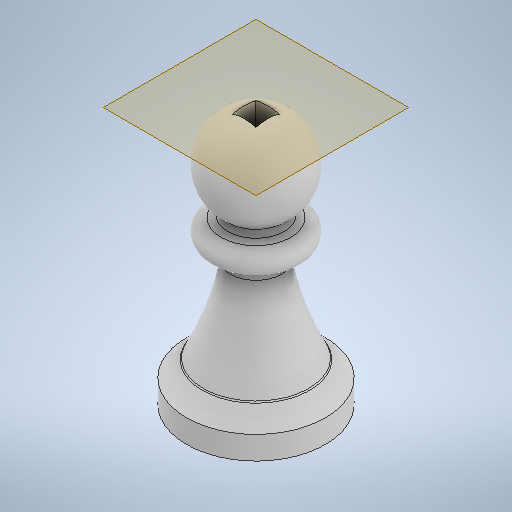
# Autodesk Inventor part: PawnUntagged
Saved by Autodesk Inventor 2025.2 (Build 292293000, 293)
## iProperties
Created: 2025-02-26
Part Number: PawnUntagged
Material: Generic
Document SubType Name: Modeling
Designer: Marcu
Density: 1 g/cm^3
Appearance: Default
Author: Marcu
Autodesk Inventor part; units mm, degrees
ref_plane "YZ Plane" through (0, 0, 0) normal (1, 0, 0) x (0, 1, 0)
ref_plane "XY Plane" through (0, 0, 0) normal (0, 0, 1) x (1, 0, 0)
sketch "Sketch1" plane through (0, 0, 0) normal (1, 0, 0) x (0, 1, 0)
  line L0 (4, 0) -> (4, 2.5)
  line L1 (4, 2.5) -> (0.0049, 2.5)
  line L2 (0.0049, 2.5) -> (0.0049, 15)
  line L3 (0.0049, 15) -> (5.0049, 15)
  line L4 (5.0049, 15) -> (8.4215, 11.5834)
  arc A0 (8.6928, 11.3905) -> (27.0718, 5.4521) centre (39.1985, 74.3936) ccw
  line L5 (30.0049, 7.9143) -> (30.0049, 7.5)
  line L6 (32.5049, 10) -> (32.5049, 10)
  line L7 (35.0049, 7.5) -> (35.0049, 7.5)
  arc A1 (55.0049, 0) -> (37.0518, 6.0621) centre (45.0049, 0) ccw
  line L8 (4, 0) -> (55.0049, 0)
  arc A2 (35.0049, 7.5) -> (35.4243, 6.1139) centre (37.5049, 7.5) ccw
  arc A3 (35.0049, 7.5) -> (32.5049, 10) centre (32.5049, 7.5) ccw
  arc A4 (32.5049, 10) -> (30.0049, 7.5) centre (32.5049, 7.5) ccw
  arc A5 (27.0718, 5.4521) -> (30.0049, 7.9143) centre (27.5049, 7.9143) ccw
  arc A6 (35.4243, 6.1139) -> (37.0518, 6.0621) centre (36.2565, 6.6683) ccw
  arc A7 (8.4215, 11.5834) -> (8.6928, 11.3905) centre (9.1286, 12.2905) ccw
  point P0 (0, 0)
  point P1 (0, 0)
  point P2 (8.5404, 11.4645)
  point P3 (30.0049, 5)
  point P4 (30.0049, 10)
  point P5 (35.0049, 10)
  point P6 (35.0049, 5)
  dimension "d0" = 4
  dimension "d1" = 2.5
  dimension "d2" = 15
  dimension "d3" = 5
  dimension "d4" = 5
  dimension "d5" = 135
  dimension "d6" = 70
  dimension "d7" = 5
  dimension "d8" = 5
  dimension "d9" = 5
  dimension "d10" = 2.5
  dimension "d11" = 1
  dimension "d12" = 1
  constraints: 18 end point, 18 point on circle, 11 tangent, 8 centre point, 7 point on line, 3 equal radius, 3 perpendicular, 2 horizontal, 2 vertical
  measures "d0" distance of point (0, 0) L8.start
  measures "d1" distance of L8.start L0.end
  measures "d2" distance of point (0, 0) L2.end
  measures "d3" distance of L2.end L3.end
  measures "d4" distance of L3.end point (8.54, 11.464)
  measures "d5" angle of L3 L4
  measures "d6" radius of A0
  measures "d7" distance of point (30.005, 5) point (30.005, 10)
  measures "d8" distance of point (30.005, 10) point (35.005, 10)
  measures "d9" distance of point (35.005, 10) point (35.005, 5)
  measures "d10" radius of A2
  measures "d11" radius of A6
  measures "d12" radius of A7
revolve "Revolution1" add sketch "Sketch1" angle 360 about axis through (0, 4, 0) along (0, 1, 0)
ref_plane "Work Plane1" through (0, 55.5625, 0) normal (0, 1, 0) x (-1, 0, 0)
sketch "Sketch2" plane through (0, 55.5625, 0) normal (0, 1, 0) x (-1, 0, 0)
  circle A0 centre (0, 0) radius 6.0621 projected
  circle A1 centre (0, 0) radius 5.4521 projected
  line L0 (2.5, 2.5) -> (2.5, -2.5)
  line L1 (-2.5, 2.5) -> (-2.5, -2.5)
  line L2 (2.5, 2.5) -> (-2.5, 2.5)
  line L3 (-2.5, -2.5) -> (2.5, -2.5)
  point P0 (0, 0)
  dimension "d18" = 2.5
  dimension "d19" = 5
  constraints: 8 end point, 2 parallel, 1 horizontal, 1 perpendicular
  measures "d18" distance from line of point (0, 0) L0
  measures "d19" distance between parallel lines of L0 L1
extrude "Extrusion1" cut sketch "Sketch2" against normal blind 7 contours L0 L3 L1 L2
body "Solid1"
